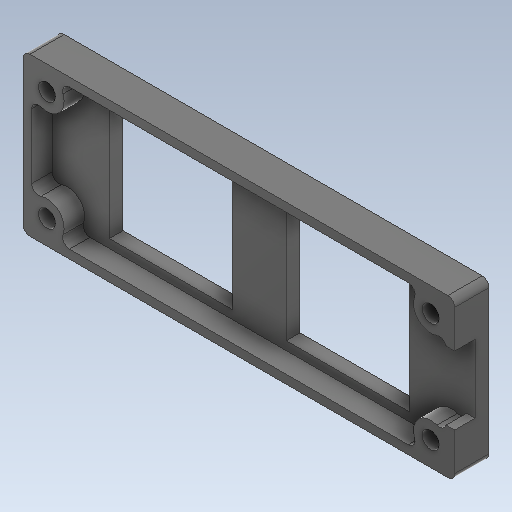
# Autodesk Inventor part: StartStopSwitch_cover_02
Saved by Autodesk Inventor 2020 (Build 240168000, 168)
## iProperties
Created: 2021-08-14
Part Number: StartStopSwitch_cover_02
Material: アセタール樹脂、黒
Document SubType Name: Modeling
Designer: Masato Kubotera
Density: 1.425 g/cm^3
Appearance: 滑らか - 黒
Mass: 3.36512 g
Surface Area: 32.6433 cm^2
Volume: 2.36149 cm^3
Author: Masato Kubotera
Title: StartStopSwitch_cover_02
Autodesk Inventor part; units mm, degrees
ref_plane "YZ Plane" through (0, 0, 0) normal (1, 0, 0) x (0, 1, 0)
ref_plane "XZ Plane" through (0, 0, 0) normal (0, 1, 0) x (-1, 0, 0)
ref_plane "XY Plane" through (0, 0, 0) normal (0, 0, 1) x (1, 0, 0)
sketch "スケッチ1" plane through (0, 0, 0) normal (0, 0, 1) x (1, 0, 0)
  line L0 (-31.5, 11.5) -> (31.5, 11.5)
  line L1 (31.5, 11.5) -> (31.5, -11.5)
  line L2 (31.5, -11.5) -> (-31.5, -11.5)
  line L3 (-31.5, -11.5) -> (-31.5, 11.5)
  line L4 (-31.5, 11.5) -> (31.5, -11.5) construction
  line L5 (31.5, 11.5) -> (-31.5, -11.5) construction
  line L6 (-30, 10) -> (30, 10) construction
  line L7 (30, 10) -> (30, -10) construction
  line L8 (30, -10) -> (-30, -10) construction
  line L9 (-30, -10) -> (-30, 10) construction
  line L10 (-30, 10) -> (30, -10) construction
  line L11 (30, 10) -> (-30, -10) construction
  circle A0 centre (-28, 8) radius 1.25
  line L12 (-31.5, 0) -> (31.5, 0) construction
  line L13 (0, 11.5) -> (0, -11.5) construction
  circle A1 centre (-28, -8) radius 1.25
  circle A2 centre (28, 8) radius 1.25
  circle A3 centre (28, -8) radius 1.25
  line L14 (-30.25, 10.25) -> (30.25, 10.25)
  line L15 (30.25, 10.25) -> (30.25, -10.25)
  line L16 (30.25, -10.25) -> (-30.25, -10.25)
  line L17 (-30.25, -10.25) -> (-30.25, 10.25)
  line L18 (-30.25, 10.25) -> (30.25, -10.25) construction
  line L19 (30.25, 10.25) -> (-30.25, -10.25) construction
  line L20 (-21.92, 9) -> (-3.92, 9)
  line L21 (-3.92, 9) -> (-3.92, -9)
  line L22 (-3.92, -9) -> (-21.92, -9)
  line L23 (-21.92, -9) -> (-21.92, 9)
  line L24 (-21.92, 9) -> (-3.92, -9) construction
  line L25 (-3.92, 9) -> (-21.92, -9) construction
  line L26 (21.92, 9) -> (3.92, 9)
  line L27 (3.92, 9) -> (3.92, -9)
  line L28 (3.92, -9) -> (21.92, -9)
  line L29 (21.92, -9) -> (21.92, 9)
  line L30 (21.92, 9) -> (3.92, -9) construction
  line L31 (3.92, 9) -> (21.92, -9) construction
  arc A4 (-30.25, 6.9103) -> (-26.9103, 10.25) centre (-28, 8) ccw
  arc A5 (-26.9103, -10.25) -> (-30.25, -6.9103) centre (-28, -8) ccw
  arc A6 (26.9103, 10.25) -> (30.25, 6.9103) centre (28, 8) ccw
  arc A7 (30.25, -6.9103) -> (26.9103, -10.25) centre (28, -8) ccw
  line L32 (30.25, 5) -> (31.5, 5)
  line L33 (30.25, -5) -> (31.5, -5)
  point P0 (0, 0)
  point P1 (0, 0)
  point P2 (-12.92, 0)
  point P3 (12.92, 0)
  point P4 (30.25, -6.9103)
  point P5 (26.9103, -10.25)
  point P6 (-30.25, -6.9103)
  point P7 (30.25, 6.9103)
  dimension "d0" = 63
  dimension "d1" = 60
  dimension "d2" = 20
  dimension "d3" = 23
  dimension "d4" = 2.5
  dimension "d5" = 2
  dimension "d6" = 2
  dimension "d7" = 20.5
  dimension "d8" = 60.5
  dimension "d17" = 18
  dimension "d18" = 18
  dimension "d19" = 17.08
  dimension "d22" = 2.5
  dimension "d23" = 10
  constraints: 68 end point, 19 symmetric about line, 16 midpoint, 8 centre point, 8 parallel, 8 point on circle, 5 horizontal, 5 point on line, 4 perpendicular, 1 coincident, 6 other
  measures "d0" distance of L1.end L2.end
  measures "d1" distance of L7.end L8.end
  measures "d2" distance of L6.end L7.end
  measures "d3" distance of L0.end L1.end
  measures "d4" diameter of A0
  measures "d5" horizontal distance of A0.centre L6.start
  measures "d6" horizontal distance of A0.centre L6.start
  measures "d7" distance of L14.end L15.end
  measures "d8" distance of L15.end L16.end
  measures "d17" distance of L21.end L22.end
  measures "d18" distance of L20.end L21.end
  measures "d19" distance from line of point (-12.92, 0) L9
  measures "d22" radius of A4
  measures "d23" distance between parallel lines of L33 L32
extrude "押し出し1" add sketch "スケッチ1" against normal blind 2
extrude "押し出し5" add sketch "スケッチ1" along normal blind 3 contours L0 L1 L32 L15 L14 L17 L16 L33 L2 L3 | A6 L14 L15 | L15 L16 A7 | A4 L17 L14 | L16 L17 A5
fillet "フィレット2" radius 1 12 edges at (-31.5, 11.5, 0.5) (-31.5, -11.5, 0.5) (31.5, -11.5, 0.5) (31.5, 11.5, 0.5) (26.9103, 10.25, 1.5) (30.25, 6.9103, 1.5) (30.25, -6.9103, 1.5) (26.9103, -10.25, 1.5) (-26.9103, -10.25, 1.5) (-30.25, -6.9103, 1.5) (-30.25, 6.9103, 1.5) (-26.9103, 10.25, 1.5)
equation "\"d6\" = d5"
equation "\"d17\" = d18"
